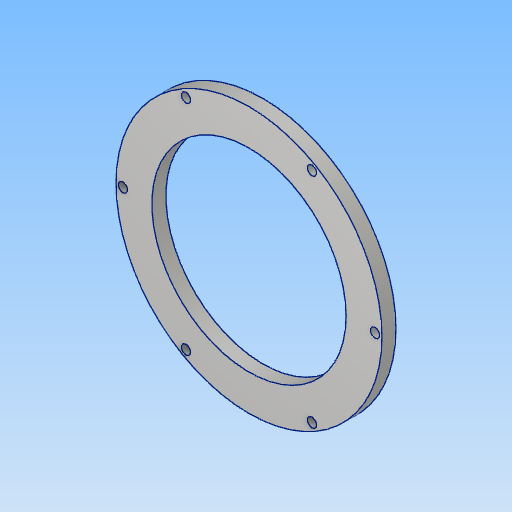
# Autodesk Inventor part: forwardBallastSealingWallDisc
Saved by Autodesk Inventor 2017 (Build 210142000, 142)
## iProperties
Created: 2016-11-26
Part Number: forwardBallastSealingWallDisc
Material: Aluminum 6061
Document SubType Name: Modeling
Designer: techn
Density: 2.7 g/cm^3
Appearance: Aluminum - Flat
Author: techn
Autodesk Inventor part; units mm, degrees
ref_plane "YZ Plane" through (0, 0, 0) normal (1, 0, 0) x (0, 1, 0)
ref_plane "XZ Plane" through (0, 0, 0) normal (0, 1, 0) x (-1, 0, 0)
ref_plane "XY Plane" through (0, 0, 0) normal (0, 0, 1) x (1, 0, 0)
sketch "Sketch1" plane through (0, 0, 0) normal (0, 0, 1) x (1, 0, 0)
  circle A0 centre (0, 0) radius 45.212
  line L0 (0, 0) -> (21.4313, 37.12)
  line L1 (0, 0) -> (42.8625, 0) construction
  circle A1 centre (21.4313, 37.12) radius 1.5875
  circle A2 centre (-21.4312, 37.12) radius 1.5875
  circle A3 centre (-42.8625, 0) radius 1.5875
  circle A4 centre (-21.4313, -37.12) radius 1.5875
  circle A5 centre (21.4312, -37.12) radius 1.5875
  circle A6 centre (42.8625, 0) radius 1.5875
  dimension "d0" = 90.424
  dimension "d1" = 42.8625
  dimension "d2" = 60
  dimension "d3" = 3.175
  dimension "d6" = 360
  constraints: 7 centre point, 4 end point, 2 coincident, 1 equal length, 1 horizontal, 13 other
  measures "d0" diameter of A0
  measures "d1" distance of L0.start L0.end
  measures "d2" angle of L1 L0
  measures "d3" diameter of A1
extrude "Extrusion1" add sketch "Sketch1" along normal blind 4.7625
sketch "Sketch2" plane through (0, 0, 4.7625) normal (0, 0, 1) x (1, 0, 0)
  circle A0 centre (0, 0) radius 33.02
  dimension "d10" = 66.04
  constraints: 1 centre point, 1 coincident
  measures "d10" diameter of A0
extrude "Extrusion2" cut sketch "Sketch2" against normal blind 25.4
body "Solid1"
